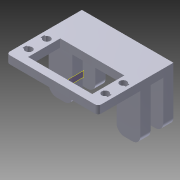
# Autodesk Inventor part: CameraCraddle
Saved by Autodesk Inventor 2014 SP1 (Build 180222100, 222)
## iProperties
Created: 2017-01-18
Part Number: CameraCraddle
Material: Generic
Document SubType Name: Modeling
Designer: danielsikar
Density: 1 g/cm^3
Appearance: Cool White
Author: danielsikar
Autodesk Inventor part; units mm, degrees
ref_plane "YZ Plane" through (0, 0, 0) normal (1, 0, 0) x (0, 1, 0)
ref_plane "XZ Plane" through (0, 0, 0) normal (0, 1, 0) x (-1, 0, 0)
sketch "Sketch1" plane through (0, 0, 0) normal (0, 0, 1) x (1, 0, 0)
  line L0 (0, 0) -> (-6.8, 0)
  line L1 (-6.8, 0) -> (-6.8, 20)
  line L2 (-6.8, 20) -> (0, 20)
  line L3 (0, 20) -> (0, 0)
  line L4 (-5.8439, 5.5) -> (-6.8, 5.5) projected
  line L5 (-6.8, 14.5) -> (-6.8, 5.5) projected
  line L6 (-6.8, 14.5) -> (-5.8439, 14.5) projected
  arc A0 (-5.8439, 14.5) -> (-5.8439, 16.9) centre (-4, 15.7) ccw projected
  line L7 (-5.8439, 16.9) -> (-6.8, 16.9) projected
  line L8 (-6.8, 20) -> (-6.8, 16.9) projected
  line L9 (0, 20) -> (-6.8, 20) projected
  line L10 (0, 0) -> (0, 20) projected
  line L11 (0, 0) -> (-6.8, 0) projected
  line L12 (-6.8, 3.1) -> (-6.8, 0) projected
  line L13 (-6.8, 3.1) -> (-5.8439, 3.1) projected
  arc A1 (-5.8439, 3.1) -> (-5.8439, 5.5) centre (-4, 4.3) ccw projected
  dimension "d0" = 6.8
  dimension "d1" = 20
  constraints: 8 end point, 2 parallel, 1 horizontal, 1 perpendicular
  measures "d0" distance of L1.end L2.end
  measures "d1" distance of L0.end L1.end
extrude "Extrusion1" add sketch "Sketch1" along normal blind 5 contours L0 L1 L13 A1 L4 L6 A0 L7 L2 L3
ref_plane "Work Plane1" through (20.15, 10, -1.65) normal (-1, 0, 0) x (0, 1, 0)
mirror "Mirror1" about plane through (20.15, 10, -1.65) normal (-1, 0, 0) of "Extrusion1"
sketch "Sketch2" plane through (-6.8, 0, 0) normal (0, -1, 0) x (1, 0, 0)
  line L0 (0, 0) -> (53.9, 0)
  line L1 (53.9, 0) -> (53.9, 5)
  line L2 (53.9, 5) -> (0, 5)
  line L3 (0, 5) -> (0, 0)
  dimension "d4" = 53.9
  constraints: 8 end point, 2 parallel, 1 horizontal, 1 perpendicular
  measures "d4" distance of L2.end L1.end
extrude "Extrusion2" add sketch "Sketch2" along normal blind 5
sketch "Sketch3" plane through (-6.8, 3.1, 0) normal (-1, 0, 0) x (0, 0, 1)
  line L0 (0, -8.1) -> (5, -8.1)
  line L1 (5, -8.1) -> (5, 16.9)
  line L2 (5, 16.9) -> (0, 16.9)
  line L3 (0, 16.9) -> (0, -8.1)
  point P0 (0, -3.1)
  dimension "d7" = 25
  constraints: 8 end point, 2 parallel, 1 horizontal, 1 perpendicular
  measures "d7" distance of L1.end L0.end
extrude "Extrusion3" add sketch "Sketch3" along normal blind 2
mirror "Mirror2" about plane through (20.15, 10, -1.65) normal (-1, 0, 0) of "Extrusion3"
fillet "Fillet1" radius 2 1 edges at (-8.8, -5, 2.5)
fillet "Fillet2" radius 2 1 edges at (49.1, -5, 2.5)
sketch "Sketch4" plane through (0, 20, 5) normal (1, 0, 0) x (0, 0, -1)
  line L0 (5, -20) -> (5, 0) projected
  line L1 (5, 0) -> (0, 0) projected
  line L2 (0, -20) -> (0, 0) projected
  line L3 (5, -20) -> (0, -20) projected
extrude "Extrusion4" cut sketch "Sketch4" against normal blind 0.25
mirror "Mirror3" about plane through (20.15, 10, -1.65) normal (-1, 0, 0) of "Extrusion4"
sketch "Sketch5" plane through (-8.8, 20, 5) normal (0, 1, 0) x (1, 0, 0)
  line L0 (0, 0) -> (57.9, 0)
  line L1 (57.9, 0) -> (57.9, 5)
  line L2 (57.9, 5) -> (0, 5)
  line L3 (0, 5) -> (0, 0)
  point P0 (8.8, 5)
  dimension "d14" = 57.9
  constraints: 8 end point, 2 parallel, 1 horizontal, 1 perpendicular
  measures "d14" distance of L2.end L1.end
extrude "Extrusion5" add sketch "Sketch5" along normal blind 5
sketch "Sketch6" plane through (-8.8, 20, 5) normal (0, -1, 0) x (1, 0, 0)
  line L0 (8.55, 0) -> (8.55, -5) projected
  line L1 (49.35, -5) -> (8.55, -5) projected
  line L2 (49.35, -5) -> (49.35, 0) projected
  line L3 (8.55, 0) -> (49.35, 0) projected
  point P0 (8.8, -5)
extrude "Extrusion6" cut sketch "Sketch6" against normal blind 0.15
sketch "Sketch7" plane through (-6.8, 0, 0) normal (0, 1, 0) x (1, 0, 0)
  line L0 (47.35, -5) -> (6.55, -5) projected
  line L1 (47.35, 0) -> (47.35, -5) projected
  line L2 (6.55, 0) -> (47.35, 0) projected
  line L3 (6.55, 0) -> (6.55, -5) projected
  point P0 (6.8, 0)
extrude "Extrusion7" cut sketch "Sketch7" against normal blind 0.15
sketch "Sketch16" plane through (-8.8, 25, 5) normal (0, 1, 0) x (1, 0, 0)
  line L0 (0, 0) -> (57.9, 0) projected
  line L1 (0, 5) -> (15, 5)
  line L2 (15, 5) -> (15, 0)
  line L3 (15, 0) -> (0, 0)
  line L4 (0, 0) -> (0, 5)
  line L5 (57.9, 5) -> (42.9, 5)
  line L6 (42.9, 5) -> (42.9, 0)
  line L7 (42.9, 0) -> (57.9, 0)
  line L8 (57.9, 0) -> (57.9, 5)
  point P0 (8.8, 5)
  dimension "d48" = 15
  dimension "d49" = 15
  constraints: 16 end point, 4 parallel, 2 horizontal, 2 perpendicular, 2 point on line
  measures "d48" distance of L2.end L3.end
  measures "d49" distance of L7.end L6.end
extrude "Extrusion13" add sketch "Sketch16" along normal blind 18
sketch "Sketch17" plane through (0, 0, 0) normal (0, 0, -1) x (-1, 0, 0)
  line L0 (8.8, -3) -> (8.8, 43) projected
  line L1 (-34.1, 25) -> (-34.1, 43) projected
  line L2 (-49.1, 43) -> (-49.1, -3) projected
  line L3 (-49.1, 43) -> (-34.1, 43)
  line L4 (-34.1, 38) -> (-34.1, 36.5)
  line L5 (-49.1, 36.5) -> (-49.1, 43)
  line L6 (-6.2, 43) -> (8.8, 43)
  line L7 (8.8, 43) -> (8.8, 38)
  line L8 (8.8, 38) -> (-6.2, 38)
  line L9 (-6.2, 38) -> (-6.2, 43)
  line L10 (-49.1, 28.15) -> (-34.1, 28.15)
  line L11 (-34.1, 28.15) -> (-34.1, 21.65)
  line L12 (-34.1, 21.65) -> (-49.1, 21.65)
  line L13 (-49.1, 21.65) -> (-49.1, 28.15)
  line L14 (-6.2, 25) -> (8.8, 25)
  line L15 (8.8, 25) -> (8.8, 30)
  line L16 (8.8, 30) -> (-6.2, 30)
  line L17 (-6.2, 30) -> (-6.2, 25)
  line L18 (-40.55, 20.15) -> (0.25, 20.15) projected
  line L19 (-49.1, 36.15) -> (-34.1, 36.15)
  line L20 (-34.1, 36.15) -> (-34.1, 42.65)
  line L21 (-34.1, 42.65) -> (-49.1, 42.65)
  line L22 (-49.1, 42.65) -> (-49.1, 36.15)
  point P0 (0, 0)
  dimension "d54" = 6.5
  dimension "d75" = 1.5
  dimension "d76" = 8
  dimension "d77" = 6.5
  constraints: 38 end point, 9 parallel, 8 point on line, 5 horizontal, 5 perpendicular
  measures "d54" distance of L10.end L11.end
  measures "d75" distance between parallel lines of L18 L12
  measures "d76" distance between parallel lines of L19 L10
  measures "d77" distance between parallel lines of L21 L19
sketch "Sketch19" plane through (-8.8, 25, 5) normal (0, 1, 0) x (1, 0, 0)
  line L0 (15, 5) -> (15, 0) projected
  line L1 (15, 0) -> (42.9, 0) projected
  line L2 (42.9, 0) -> (42.9, 5) projected
  line L3 (42.9, 5) -> (15, 5) projected
  point P0 (8.8, 5)
extrude "Extrusion17" add sketch "Sketch19" along normal up to surface (18 mm away)
extrude "Extrusion18" add sketch "Sketch17" along normal blind 30 contours L11 L12 L2 L10 L1 | L19 L2 L21 L1
fillet "Fillet16" radius 5 4 edges at (49.1, 39.4, -30) (34.1, 39.4, -30) (34.1, 24.9, -30) (49.1, 24.9, -30)
mirror "Mirror6" about plane through (20.15, 10, -1.65) normal (-1, 0, 0) of "Extrusion18", "Mirror1"
sketch "Sketch20" plane through (-8.8, 43, 5) normal (0, 1, 0) x (1, 0, 0)
  line L0 (57.9, 5) -> (0, 5) projected
  line L1 (0, 5) -> (0, 0) projected
  line L2 (0, 0) -> (57.9, 0) projected
  line L3 (57.9, 0) -> (57.9, 5) projected
  point P0 (8.8, 5)
extrude "Extrusion19" cut sketch "Sketch20" against normal up to surface (0.35 mm away)
mirror "Mirror7" about plane through (20.15, 10, -1.65) normal (-1, 0, 0) of "Fillet16"
ref_plane "Work Plane2" through (20.15, 10, -1.65) normal (-1, 0, 0) x (0, 1, 0)
ref_plane "Work Plane3" through (20.15, 10, -1.65) normal (-1, 0, 0) x (0, 1, 0)
body "Solid1"
